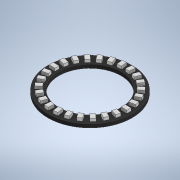
# Autodesk Inventor part: ledRing
Saved by Autodesk Inventor 2020 (Build 240168000, 168)
## iProperties
Created: 2020-02-08
Part Number: ledRing
Material: Generic
Document SubType Name: Modeling
Designer: Chris Gerth
Density: 1 g/cm^3
Appearance: Default
Author: Chris Gerth
Autodesk Inventor part; units mm, degrees
ref_plane "YZ Plane" through (0, 0, 0) normal (1, 0, 0) x (0, 1, 0)
ref_plane "XZ Plane" through (0, 0, 0) normal (0, 1, 0) x (-1, 0, 0)
ref_plane "XY Plane" through (0, 0, 0) normal (0, 0, 1) x (1, 0, 0)
sketch "Sketch1" plane through (0, 0, 0) normal (0, 1, 0) x (-1, 0, 0)
  circle A0 centre (0, 0) radius 22.352
  circle A1 centre (0, 0) radius 30.226
  dimension "d0" = 44.704
  dimension "d1" = 60.452
  constraints: 2 centre point, 2 coincident
  measures "d0" diameter of A0
  measures "d1" diameter of A1
extrude "Extrusion1" add sketch "Sketch1" along normal blind 2.54
sketch "Sketch2" plane through (0, 2.54, 0) normal (0, 1, 0) x (1, 0, 0)
  line L0 (-28.152, -1.3552) -> (-23.9586, -1.3552)
  line L1 (-23.9586, -1.3552) -> (-23.9586, 1.7132)
  line L2 (-23.9586, 1.7132) -> (-28.152, 1.7132)
  line L3 (-28.152, 1.7132) -> (-28.152, -1.3552)
  line L4 (-27.7439, -5.0738) -> (-27.0096, -8.053)
  line L5 (-23.6724, -4.0703) -> (-27.7439, -5.0738)
  line L6 (-22.9381, -7.0495) -> (-23.6724, -4.0703)
  line L7 (-27.0096, -8.053) -> (-22.9381, -7.0495)
  line L8 (-25.7235, -11.566) -> (-24.2975, -14.2828)
  line L9 (-22.0104, -9.6172) -> (-25.7235, -11.566)
  line L10 (-20.5845, -12.3341) -> (-22.0104, -9.6172)
  line L11 (-24.2975, -14.2828) -> (-20.5845, -12.3341)
  line L12 (-22.2081, -17.3859) -> (-20.1734, -19.6826)
  line L13 (-19.0693, -14.6052) -> (-22.2081, -17.3859)
  line L14 (-17.0346, -16.9018) -> (-19.0693, -14.6052)
  line L15 (-20.1734, -19.6826) -> (-17.0346, -16.9018)
  line L16 (-17.402, -22.1954) -> (-14.8768, -23.9384)
  line L17 (-15.0199, -18.7443) -> (-17.402, -22.1954)
  line L18 (-12.4947, -20.4874) -> (-15.0199, -18.7443)
  line L19 (-14.8768, -23.9384) -> (-12.4947, -20.4874)
  line L20 (-11.5847, -25.7151) -> (-8.7157, -26.8031)
  line L21 (-10.0977, -21.7942) -> (-11.5847, -25.7151)
  line L22 (-7.2287, -22.8822) -> (-10.0977, -21.7942)
  line L23 (-8.7157, -26.8031) -> (-7.2287, -22.8822)
  line L24 (-5.094, -27.7402) -> (-2.048, -28.1101)
  line L25 (-4.5886, -23.5774) -> (-5.094, -27.7402)
  line L26 (-1.5426, -23.9472) -> (-4.5886, -23.5774)
  line L27 (-2.048, -28.1101) -> (-1.5426, -23.9472)
  line L28 (1.6927, -28.1532) -> (4.7386, -27.7834)
  line L29 (1.1872, -23.9904) -> (1.6927, -28.1532)
  line L30 (4.2332, -23.6205) -> (1.1872, -23.9904)
  line L31 (4.7386, -27.7834) -> (4.2332, -23.6205)
  line L32 (8.381, -26.93) -> (11.2499, -25.842)
  line L33 (6.894, -23.0092) -> (8.381, -26.93)
  line L34 (9.7629, -21.9211) -> (6.894, -23.0092)
  line L35 (11.2499, -25.842) -> (9.7629, -21.9211)
  line L36 (14.5822, -24.1418) -> (17.1074, -22.3988)
  line L37 (12.2001, -20.6907) -> (14.5822, -24.1418)
  line L38 (14.7253, -18.9477) -> (12.2001, -20.6907)
  line L39 (17.1074, -22.3988) -> (14.7253, -18.9477)
  line L40 (19.936, -19.9505) -> (21.9707, -17.6538)
  line L41 (16.7972, -17.1698) -> (19.936, -19.9505)
  line L42 (18.8319, -14.8731) -> (16.7972, -17.1698)
  line L43 (21.9707, -17.6538) -> (18.8319, -14.8731)
  line L44 (24.1312, -14.5998) -> (25.5571, -11.8829)
  line L45 (20.4181, -12.651) -> (24.1312, -14.5998)
  line L46 (21.8441, -9.9342) -> (20.4181, -12.651)
  line L47 (25.5571, -11.8829) -> (21.8441, -9.9342)
  line L48 (26.9239, -8.4006) -> (27.6582, -5.4214)
  line L49 (22.8524, -7.397) -> (26.9239, -8.4006)
  line L50 (23.5867, -4.4179) -> (22.8524, -7.397)
  line L51 (27.6582, -5.4214) -> (23.5867, -4.4179)
  line L52 (28.152, -1.7132) -> (28.152, 1.3552)
  line L53 (23.9586, -1.7132) -> (28.152, -1.7132)
  line L54 (23.9586, 1.3552) -> (23.9586, -1.7132)
  line L55 (28.152, 1.3552) -> (23.9586, 1.3552)
  line L56 (27.7439, 5.0738) -> (27.0096, 8.053)
  line L57 (23.6724, 4.0703) -> (27.7439, 5.0738)
  line L58 (22.9381, 7.0495) -> (23.6724, 4.0703)
  line L59 (27.0096, 8.053) -> (22.9381, 7.0495)
  line L60 (25.7235, 11.566) -> (24.2975, 14.2828)
  line L61 (22.0104, 9.6172) -> (25.7235, 11.566)
  line L62 (20.5845, 12.3341) -> (22.0104, 9.6172)
  line L63 (24.2975, 14.2828) -> (20.5845, 12.3341)
  line L64 (22.2081, 17.3859) -> (20.1734, 19.6826)
  line L65 (19.0693, 14.6052) -> (22.2081, 17.3859)
  line L66 (17.0346, 16.9018) -> (19.0693, 14.6052)
  line L67 (20.1734, 19.6826) -> (17.0346, 16.9018)
  line L68 (17.402, 22.1954) -> (14.8768, 23.9384)
  line L69 (15.0199, 18.7443) -> (17.402, 22.1954)
  line L70 (12.4947, 20.4874) -> (15.0199, 18.7443)
  line L71 (14.8768, 23.9384) -> (12.4947, 20.4874)
  line L72 (11.5847, 25.7151) -> (8.7157, 26.8031)
  line L73 (10.0977, 21.7942) -> (11.5847, 25.7151)
  line L74 (7.2287, 22.8822) -> (10.0977, 21.7942)
  line L75 (8.7157, 26.8031) -> (7.2287, 22.8822)
  line L76 (5.094, 27.7402) -> (2.048, 28.1101)
  line L77 (4.5886, 23.5774) -> (5.094, 27.7402)
  line L78 (1.5426, 23.9472) -> (4.5886, 23.5774)
  line L79 (2.048, 28.1101) -> (1.5426, 23.9472)
  line L80 (-1.6927, 28.1532) -> (-4.7386, 27.7834)
  line L81 (-1.1872, 23.9904) -> (-1.6927, 28.1532)
  line L82 (-4.2332, 23.6205) -> (-1.1872, 23.9904)
  line L83 (-4.7386, 27.7834) -> (-4.2332, 23.6205)
  line L84 (-8.381, 26.93) -> (-11.2499, 25.842)
  line L85 (-6.894, 23.0092) -> (-8.381, 26.93)
  line L86 (-9.7629, 21.9211) -> (-6.894, 23.0092)
  line L87 (-11.2499, 25.842) -> (-9.7629, 21.9211)
  line L88 (-14.5822, 24.1418) -> (-17.1074, 22.3988)
  line L89 (-12.2001, 20.6907) -> (-14.5822, 24.1418)
  line L90 (-14.7253, 18.9477) -> (-12.2001, 20.6907)
  line L91 (-17.1074, 22.3988) -> (-14.7253, 18.9477)
  line L92 (-19.936, 19.9505) -> (-21.9707, 17.6538)
  line L93 (-16.7972, 17.1698) -> (-19.936, 19.9505)
  line L94 (-18.8319, 14.8731) -> (-16.7972, 17.1698)
  line L95 (-21.9707, 17.6538) -> (-18.8319, 14.8731)
  line L96 (-24.1312, 14.5998) -> (-25.5571, 11.8829)
  line L97 (-20.4181, 12.651) -> (-24.1312, 14.5998)
  line L98 (-21.8441, 9.9342) -> (-20.4181, 12.651)
  line L99 (-25.5571, 11.8829) -> (-21.8441, 9.9342)
  line L100 (-26.9239, 8.4006) -> (-27.6582, 5.4214)
  line L101 (-22.8524, 7.397) -> (-26.9239, 8.4006)
  line L102 (-23.5867, 4.4179) -> (-22.8524, 7.397)
  line L103 (-27.6582, 5.4214) -> (-23.5867, 4.4179)
  point P0 (0, 0)
  dimension "d6" = 360
  constraints: 208 end point, 2 parallel, 1 horizontal, 1 perpendicular, 209 other
extrude "Extrusion2" add sketch "Sketch2" along normal blind 2.032
body "Solid1"
